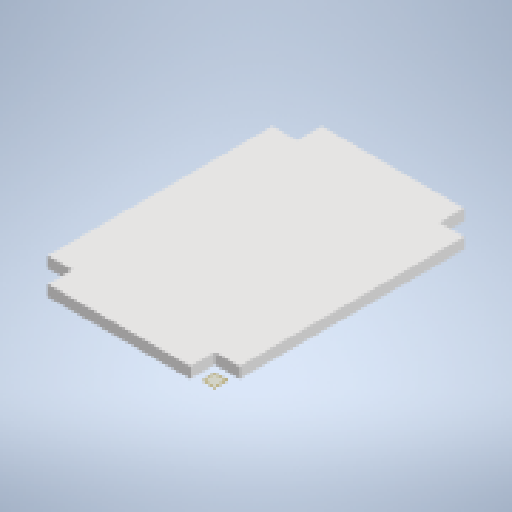
# Autodesk Inventor part: Shelf
Saved by Autodesk Inventor 2024 (Build 280153000, 153)
## iProperties
Created: 2025-09-20
Part Number: Shelf
Material: Generic
Document SubType Name: Modeling
Designer: Emil
Density: 1 g/cm^3
Appearance: Default
Author: Emil
Autodesk Inventor part; units mm, degrees
ref_plane "YZ Plane" through (0, 0, 0) normal (1, 0, 0) x (0, 1, 0)
ref_plane "XZ Plane" through (0, 0, 0) normal (0, 1, 0) x (-1, 0, 0)
ref_plane "XY Plane" through (0, 0, 0) normal (0, 0, 1) x (1, 0, 0)
sketch "Sketch2" plane through (0, 0, 0) normal (0, 1, 0) x (-1, 0, 0)
  line L0 (0, 0) -> (350, 0)
  line L1 (350, 0) -> (350, -500)
  line L2 (350, -500) -> (0, -500)
  line L3 (0, -500) -> (0, 0)
  line L4 (350, 0) -> (305, 0)
  line L5 (305, 0) -> (305, -45)
  line L6 (305, -45) -> (350, -45)
  line L7 (350, -45) -> (350, 0)
  line L8 (350, -500) -> (305, -500)
  line L9 (305, -500) -> (305, -455)
  line L10 (305, -455) -> (350, -455)
  line L11 (350, -455) -> (350, -500)
  line L12 (0, -500) -> (45, -500)
  line L13 (45, -500) -> (45, -455)
  line L14 (45, -455) -> (0, -455)
  line L15 (0, -455) -> (0, -500)
  line L16 (0, 0) -> (45, 0)
  line L17 (45, 0) -> (45, -45)
  line L18 (45, -45) -> (0, -45)
  line L19 (0, -45) -> (0, 0)
  point P0 (0, -45)
  point P1 (0, -455)
  point P2 (350, -455)
  point P3 (350, -45)
  point P4 (305, 0)
  point P5 (45, 0)
  dimension "d0" = 350
  dimension "d1" = 500
  dimension "d12" = 45
  dimension "d13" = 45
  dimension "d14" = 45
  dimension "d15" = 45
  dimension "d16" = 45
  dimension "d17" = 45
  dimension "d18" = 45
  dimension "d19" = 45
  constraints: 40 end point, 10 parallel, 5 horizontal, 5 perpendicular
  measures "d0" distance of L1.end L2.end
  measures "d1" distance of L0.end L1.end
  measures "d12" distance of L6.end L5.end
  measures "d13" distance of L5.end L4.end
  measures "d14" distance of L9.end L10.end
  measures "d15" distance of L8.end L9.end
  measures "d16" distance of L14.end L13.end
  measures "d17" distance of L13.end L12.end
  measures "d18" distance of L17.end L18.end
  measures "d19" distance of L16.end L17.end
ref_plane "Work Plane1" through (0, 20, 0) normal (0, 1, 0) x (1, 0, 0)
extrude "Extrusion2" add sketch "Sketch2" along normal blind 20 contours L0 L5 L6 L1 L10 L9 L2 L13 L14 L3 L18 L17
body "Solid2"
